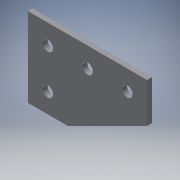
# Autodesk Inventor part: bottom gusset
Saved by Autodesk Inventor 2016 (Build 200138000, 138)
## iProperties
Created: 2016-04-20
Part Number: bottom gusset
Material: Generic
Document SubType Name: Modeling
Designer: gus
Density: 1 g/cm^3
Appearance: Default
Author: gus
Autodesk Inventor part; units mm, degrees
ref_plane "YZ Plane" through (0, 0, 0) normal (1, 0, 0) x (0, 1, 0)
ref_plane "XZ Plane" through (0, 0, 0) normal (0, 1, 0) x (-1, 0, 0)
ref_plane "XY Plane" through (0, 0, 0) normal (0, 0, 1) x (1, 0, 0)
sketch "Sketch1" plane through (0, 0, 0) normal (0, 0, 1) x (1, 0, 0)
  line L0 (0, 0) -> (76.2, 0)
  line L1 (76.2, 0) -> (76.2, -25.4)
  line L2 (76.2, -25.4) -> (25.4, -50.8)
  line L3 (25.4, -50.8) -> (0, -50.8)
  line L4 (0, -50.8) -> (0, 0)
  circle A0 centre (63.5, -12.7) radius 3.3734
  circle A1 centre (38.1, -12.7) radius 3.3734
  circle A2 centre (12.7, -12.7) radius 3.3734
  circle A3 centre (12.7, -38.1) radius 3.3734
  dimension "d0" = 25.4
  dimension "d1" = 25.4
  dimension "d2" = 76.2
  dimension "d3" = 50.8
  dimension "d4" = 6.7469
  dimension "d5" = 12.7
  dimension "d6" = 12.7
  dimension "d7" = 12.7
  dimension "d8" = 12.7
  dimension "d9" = 12.7
  dimension "d10" = 38.1
  dimension "d11" = 12.7
  dimension "d12" = 12.7
  constraints: 10 end point, 4 centre point, 3 equal radius, 2 perpendicular, 1 horizontal, 1 parallel
  measures "d0" distance of L0.end L1.end
  measures "d1" distance of L2.end L3.end
  measures "d2" distance of L0.start L0.end
  measures "d3" distance of L3.end L0.start
  measures "d4" diameter of A0
  measures "d5" distance from line of L0 A0.centre
  measures "d6" distance from line of L0 A1.centre
  measures "d7" distance from line of L0 A2.centre
  measures "d8" distance from line of A2.centre L4
  measures "d9" distance from line of A3.centre L4
  measures "d10" distance from line of L1 A1.centre
  measures "d11" distance from line of A0.centre L1
  measures "d12" distance from line of L3 A3.centre
extrude "Extrusion1" add sketch "Sketch1" along normal blind 3.175
body "Solid1"
